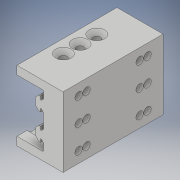
# Autodesk Inventor part: NerfRailMount
Saved by Autodesk Inventor 2018.3 (Build 223284000, 284)
## iProperties
Created: 2019-08-17
Part Number: NerfRailMount
Material: Generic
Document SubType Name: Modeling
Designer: Srinity
Density: 1 g/cm^3
Appearance: Default
Author: Srinity
Autodesk Inventor part; units mm, degrees
ref_plane "YZ Plane" through (0, 0, 0) normal (1, 0, 0) x (0, 1, 0)
ref_plane "XZ Plane" through (0, 0, 0) normal (0, 1, 0) x (-1, 0, 0)
ref_plane "XY Plane" through (0, 0, 0) normal (0, 0, 1) x (1, 0, 0)
sketch "Sketch1" plane through (0, 0, 0) normal (0, 0, 1) x (1, 0, 0)
  line L0 (3.69, 10) -> (3.9, 9.79)
  line L1 (3.69, 10) -> (3.9, 10.21)
  line L2 (3.9, 10.21) -> (3.9, 12.8393)
  line L3 (3.9, 12.8393) -> (6.5607, 15.5)
  line L4 (6.5607, 15.5) -> (8.2, 15.5)
  line L5 (8.2, 15.5) -> (8.2, 13.125)
  line L6 (8.2, 13.125) -> (8.545, 13.125)
  line L7 (8.545, 13.125) -> (10, 14.58)
  line L8 (10, 14.58) -> (10, 19.5)
  arc A0 (10, 19.5) -> (9.5, 20) centre (9.5, 19.5) ccw
  line L9 (9.5, 20) -> (4.58, 20)
  line L10 (3.125, 18.545) -> (4.58, 20)
  line L11 (3.125, 18.2) -> (3.125, 18.545)
  line L12 (5.5, 18.2) -> (3.125, 18.2)
  line L13 (5.5, 16.5607) -> (5.5, 18.2)
  line L14 (2.8393, 13.9) -> (5.5, 16.5607)
  line L15 (0.21, 13.9) -> (2.8393, 13.9)
  line L16 (0, 13.69) -> (0.21, 13.9)
  line L17 (0, 13.69) -> (-0.21, 13.9)
  line L18 (-0.21, 13.9) -> (-2.8393, 13.9)
  line L19 (-2.8393, 13.9) -> (-5.5, 16.5607)
  line L20 (-5.5, 16.5607) -> (-5.5, 18.2)
  line L21 (-5.5, 18.2) -> (-3.125, 18.2)
  line L22 (-3.125, 18.2) -> (-3.125, 18.545)
  line L23 (-3.125, 18.545) -> (-4.58, 20)
  line L24 (-4.58, 20) -> (-9.5, 20)
  arc A1 (-9.5, 20) -> (-10, 19.5) centre (-9.5, 19.5) ccw
  line L25 (-10, 14.58) -> (-10, 19.5)
  line L26 (-8.545, 13.125) -> (-10, 14.58)
  line L27 (-8.2, 13.125) -> (-8.545, 13.125)
  line L28 (-8.2, 15.5) -> (-8.2, 13.125)
  line L29 (-6.5607, 15.5) -> (-8.2, 15.5)
  line L30 (-3.9, 12.8393) -> (-6.5607, 15.5)
  line L31 (-3.9, 10.21) -> (-3.9, 12.8393)
  line L32 (-3.69, 10) -> (-3.9, 10.21)
  line L33 (-3.69, 10) -> (-3.9, 9.79)
  line L34 (-3.9, 9.79) -> (-3.9, 7.1607)
  line L35 (-3.9, 7.1607) -> (-6.5607, 4.5)
  line L36 (-6.5607, 4.5) -> (-8.2, 4.5)
  line L37 (-8.2, 4.5) -> (-8.2, 6.875)
  line L38 (-8.2, 6.875) -> (-8.545, 6.875)
  line L39 (-8.545, 6.875) -> (-10, 5.42)
  line L40 (-10, -5.42) -> (-10, 5.42)
  line L41 (-8.545, -6.875) -> (-10, -5.42)
  line L42 (-8.2, -6.875) -> (-8.545, -6.875)
  line L43 (-8.2, -4.5) -> (-8.2, -6.875)
  line L44 (-6.5607, -4.5) -> (-8.2, -4.5)
  line L45 (-3.9, -7.1607) -> (-6.5607, -4.5)
  line L46 (-3.9, -9.79) -> (-3.9, -7.1607)
  line L47 (-3.69, -10) -> (-3.9, -9.79)
  line L48 (-3.69, -10) -> (-3.9, -10.21)
  line L49 (-3.9, -10.21) -> (-3.9, -12.8393)
  line L50 (-3.9, -12.8393) -> (-6.5607, -15.5)
  line L51 (-6.5607, -15.5) -> (-8.2, -15.5)
  line L52 (-8.2, -15.5) -> (-8.2, -13.125)
  line L53 (-8.2, -13.125) -> (-8.545, -13.125)
  line L54 (-8.545, -13.125) -> (-10, -14.58)
  line L55 (-10, -19.5) -> (-10, -14.58)
  arc A2 (-10, -19.5) -> (-9.5, -20) centre (-9.5, -19.5) ccw
  line L56 (-4.58, -20) -> (-9.5, -20)
  line L57 (-3.125, -18.545) -> (-4.58, -20)
  line L58 (-3.125, -18.2) -> (-3.125, -18.545)
  line L59 (-5.5, -18.2) -> (-3.125, -18.2)
  line L60 (-5.5, -16.5607) -> (-5.5, -18.2)
  line L61 (-2.8393, -13.9) -> (-5.5, -16.5607)
  line L62 (-0.21, -13.9) -> (-2.8393, -13.9)
  line L63 (0, -13.69) -> (-0.21, -13.9)
  line L64 (0, -13.69) -> (0.21, -13.9)
  line L65 (0.21, -13.9) -> (2.8393, -13.9)
  line L66 (2.8393, -13.9) -> (5.5, -16.5607)
  line L67 (5.5, -16.5607) -> (5.5, -18.2)
  line L68 (5.5, -18.2) -> (3.125, -18.2)
  line L69 (3.125, -18.2) -> (3.125, -18.545)
  line L70 (3.125, -18.545) -> (4.58, -20)
  line L71 (9.5, -20) -> (4.58, -20)
  arc A3 (9.5, -20) -> (10, -19.5) centre (9.5, -19.5) ccw
  line L72 (10, -19.5) -> (10, -14.58)
  line L73 (8.545, -13.125) -> (10, -14.58)
  line L74 (8.2, -13.125) -> (8.545, -13.125)
  line L75 (8.2, -15.5) -> (8.2, -13.125)
  line L76 (6.5607, -15.5) -> (8.2, -15.5)
  line L77 (3.9, -12.8393) -> (6.5607, -15.5)
  line L78 (3.9, -10.21) -> (3.9, -12.8393)
  line L79 (3.69, -10) -> (3.9, -10.21)
  line L80 (3.69, -10) -> (3.9, -9.79)
  line L81 (3.9, -9.79) -> (3.9, -7.1607)
  line L82 (3.9, -7.1607) -> (6.5607, -4.5)
  line L83 (6.5607, -4.5) -> (8.2, -4.5)
  line L84 (8.2, -4.5) -> (8.2, -6.875)
  line L85 (8.2, -6.875) -> (8.545, -6.875)
  line L86 (8.545, -6.875) -> (10, -5.42)
  line L87 (10, -5.42) -> (10, 5.42)
  line L88 (8.545, 6.875) -> (10, 5.42)
  line L89 (8.2, 6.875) -> (8.545, 6.875)
  line L90 (8.2, 4.5) -> (8.2, 6.875)
  line L91 (6.5607, 4.5) -> (8.2, 4.5)
  line L92 (3.9, 7.1607) -> (6.5607, 4.5)
  line L93 (3.9, 9.79) -> (3.9, 7.1607)
  circle A4 centre (0, -10) radius 2.1
  circle A5 centre (0, 10) radius 2.1
  line L94 (-8.2, -2.7) -> (-6.2393, -2.7)
  line L95 (-8.2, -2.7) -> (-8.2, 2.7)
  line L96 (-8.2, 2.7) -> (-6.2393, 2.7)
  line L97 (-6.2393, 2.7) -> (-2.8393, 6.1)
  line L98 (-2.8393, 6.1) -> (2.8393, 6.1)
  line L99 (6.2393, 2.7) -> (2.8393, 6.1)
  line L100 (8.2, 2.7) -> (6.2393, 2.7)
  line L101 (8.2, -2.7) -> (8.2, 2.7)
  line L102 (8.2, -2.7) -> (6.2393, -2.7)
  line L103 (6.2393, -2.7) -> (2.8393, -6.1)
  line L104 (-2.8393, -6.1) -> (2.8393, -6.1)
  line L105 (-6.2393, -2.7) -> (-2.8393, -6.1)
  line L106 (10.25, 19.5) -> (10.25, 14.4764)
  line L107 (10.25, 14.4764) -> (8.6486, 12.875)
  line L108 (8.6486, 12.875) -> (7.95, 12.875)
  line L109 (7.95, 12.875) -> (7.95, 15.25)
  line L110 (7.95, 15.25) -> (6.6642, 15.25)
  line L111 (6.6642, 15.25) -> (4.15, 12.7358)
  line L112 (4.15, 12.7358) -> (4.15, 10.1064)
  line L113 (4.15, 9.8936) -> (4.15, 7.2642)
  line L114 (4.15, 7.2642) -> (6.6642, 4.75)
  line L115 (6.6642, 4.75) -> (7.95, 4.75)
  line L116 (7.95, 4.75) -> (7.95, 7.125)
  line L117 (7.95, 7.125) -> (8.6486, 7.125)
  line L118 (8.6486, 7.125) -> (10.25, 5.5236)
  line L119 (10.25, 5.5236) -> (10.25, -5.5236)
  line L120 (10.25, -5.5236) -> (8.6486, -7.125)
  line L121 (8.6486, -7.125) -> (7.95, -7.125)
  line L122 (7.95, -7.125) -> (7.95, -4.75)
  line L123 (7.95, -4.75) -> (6.6642, -4.75)
  line L124 (6.6642, -4.75) -> (4.15, -7.2642)
  line L125 (4.15, -7.2642) -> (4.15, -9.8936)
  line L126 (4.15, -10.1064) -> (4.15, -12.7358)
  line L127 (4.15, -12.7358) -> (6.6642, -15.25)
  line L128 (6.6642, -15.25) -> (7.95, -15.25)
  line L129 (7.95, -15.25) -> (7.95, -12.875)
  line L130 (7.95, -12.875) -> (8.6486, -12.875)
  line L131 (8.6486, -12.875) -> (10.25, -14.4764)
  line L132 (10.25, -14.4764) -> (10.25, -19.5)
  arc A6 (9.5, -20.25) -> (10.25, -19.5) centre (9.5, -19.5) ccw
  line L133 (9.5, -20.25) -> (-10, -20.25)
  line L134 (4.4764, 20.25) -> (9.5, 20.25)
  arc A7 (10.25, 19.5) -> (9.5, 20.25) centre (9.5, 19.5) ccw
  line L135 (4.15, 10.1064) -> (4.15, 9.8936)
  line L136 (4.15, -9.8936) -> (4.15, -10.1064)
  line L137 (-10, 20.25) -> (-10, 26.6)
  line L138 (-10, 26.6) -> (25.0836, 26.6)
  line L139 (25.0836, 26.6) -> (25.0836, -26.6)
  line L140 (25.0836, -26.6) -> (-10, -26.6)
  line L141 (-10, -26.6) -> (-10, -20.25)
  line L142 (25.0836, -21.0887) -> (25.0836, 18.3413)
  line L143 (4.4764, 20.25) -> (-10, 20.25)
  point P0 (0, 0)
  dimension "d0" = 0.25
  dimension "d1" = 6.35
  dimension "d2" = 6.35
  dimension "d27" = 14.8336
  dimension "d28" = 20.25
  constraints: 288 end point, 12 point on circle, 8 centre point, 5 vertical, 3 collinear, 3 perpendicular, 1 horizontal, 1 tangent, 27 other
  measures "d0" distance between parallel lines of L87 L119
  measures "d1" distance between parallel lines of L138 L134
  measures "d2" distance between parallel lines of L140 L133
  measures "d27" distance between parallel lines of L142 L119
  measures "d28" distance between parallel lines of L137 L106
extrude "Extrusion1" add sketch "Sketch1" against normal blind 76.2 contours A7 L134 L143 L137 L138 L139 L140 L141 L133 A6 L132 L131 L130 L129 L128 L127 L126 L136 L125 L124 L123 L122 L121 L120 L119 L118 L117 L116 L115 L114 L113 L135 L112 L111 L110 L109 L108 L107 L106
sketch "Sketch2" plane through (-10, -26.6, 0) normal (0, -1, 0) x (1, 0, 0)
  circle A0 centre (10, -25.4) radius 2.75
  circle A1 centre (10, -38.1) radius 2.75
  circle A2 centre (10, -50.8) radius 2.75
  point P0 (10, 0)
  dimension "d5" = 5.5
  dimension "d6" = 12.7
  dimension "d7" = 12.7
  dimension "d8" = 25.4
  constraints: 3 centre point, 3 vertical alignment, 2 equal radius
  measures "d5" diameter of A0
  measures "d6" distance of A1.centre A0.centre
  measures "d7" distance of A2.centre A1.centre
  measures "d8" distance of point (10, 0) A0.centre
extrude "Extrusion2" cut sketch "Sketch2" against normal through all
sketch "Sketch5" plane through (25.0836, -26.6, 0) normal (1, 0, 0) x (0, 0, -1)
  circle A0 centre (11.85, 26.6) radius 2.794
  circle A1 centre (11.85, 44.675) radius 2.794
  circle A2 centre (11.85, 8.525) radius 2.794
  circle A3 centre (17.85, 26.6) radius 2.794
  circle A4 centre (17.85, 44.675) radius 2.794
  circle A5 centre (17.85, 8.525) radius 2.794
  circle A6 centre (58.35, 26.6) radius 2.794
  circle A7 centre (58.35, 44.675) radius 2.794
  circle A8 centre (58.35, 8.525) radius 2.794
  circle A9 centre (64.35, 26.6) radius 2.794
  circle A10 centre (64.35, 44.675) radius 2.794
  circle A11 centre (64.35, 8.525) radius 2.794
  line L0 (0, 0) -> (0, 53.2) projected
  line L1 (38.1, 36.6351) -> (38.1, 5.7689)
  point P0 (0, 26.6)
  point P1 (0, 26.6)
  dimension "d14" = 5.588
  dimension "d15" = 52.5
  dimension "d16" = 40.5
  dimension "d17" = 38.1
  dimension "d18" = 20.25
  dimension "d19" = 26.25
  dimension "d22" = 18.075
  dimension "d23" = 18.075
  constraints: 12 centre point, 11 equal radius, 10 horizontal alignment, 8 vertical alignment, 2 end point, 1 midpoint, 1 vertical
  measures "d14" diameter of A0
  measures "d15" distance of A9.centre A0.centre
  measures "d16" distance of A3.centre A6.centre
  measures "d17" distance between parallel lines of L0 L1
  measures "d18" distance from line of L1 A6.centre
  measures "d19" distance from line of L1 A9.centre
  measures "d22" distance of A9.centre A11.centre
  measures "d23" distance of A10.centre A9.centre
extrude "Extrusion4" cut sketch "Sketch5" against normal through all
sketch "Sketch6" plane through (-10, -26.6, 0) normal (-1, 0, 0) x (0, 0, 1)
  circle A0 centre (-11.85, 8.525) radius 2.794 construction
  circle A1 centre (-11.85, 8.525) radius 4.7625
  circle A2 centre (-17.85, 8.525) radius 2.794 construction
  circle A3 centre (-17.85, 8.525) radius 4.7625
  circle A4 centre (-17.85, 26.6) radius 2.794 construction
  circle A5 centre (-17.85, 26.6) radius 4.7625
  circle A6 centre (-11.85, 26.6) radius 2.794 construction
  circle A7 centre (-11.85, 26.6) radius 4.7625
  circle A8 centre (-11.85, 44.675) radius 2.794 construction
  circle A9 centre (-11.85, 44.675) radius 4.7625
  arc A10 (-20.2533, 46.1) -> (-15.4467, 46.1) centre (-17.85, 44.675) ccw construction
  circle A11 centre (-17.85, 44.675) radius 4.7625
  arc A12 (-55.9467, 7.1) -> (-60.7533, 7.1) centre (-58.35, 8.525) ccw construction
  circle A13 centre (-58.35, 8.525) radius 4.7625
  arc A14 (-61.9467, 7.1) -> (-66.7533, 7.1) centre (-64.35, 8.525) ccw construction
  circle A15 centre (-64.35, 8.525) radius 4.7625
  circle A16 centre (-58.35, 26.6) radius 2.794 construction
  circle A17 centre (-58.35, 26.6) radius 4.7625
  circle A18 centre (-64.35, 26.6) radius 2.794 construction
  circle A19 centre (-64.35, 26.6) radius 4.7625
  circle A20 centre (-64.35, 44.675) radius 2.794 construction
  circle A21 centre (-64.35, 44.675) radius 4.7625
  circle A22 centre (-58.35, 44.675) radius 2.794 construction
  circle A23 centre (-58.35, 44.675) radius 4.7625
  point P0 (0, 26.6)
  dimension "d24" = 9.525
  constraints: 12 centre point, 12 coincident, 11 equal radius
  measures "d24" diameter of A1
extrude "Extrusion5" cut sketch "Sketch6" against normal blind 26.6
chamfer "Chamfer1" distance 3.175 angle 45 6 edges at (-2.75, -26.6, -50.8) (-2.75, -26.6, -38.1) (-2.75, -26.6, -25.4) (-2.75, 26.6, -25.4) (-2.75, 26.6, -38.1) (-2.75, 26.6, -50.8)
equation "\"d2\" = d1"
equation "\"d7\" = d6"
equation "\"d18\" = 0.5 * d16"
equation "\"d19\" = 0.5 * d15"
body "Solid1"
